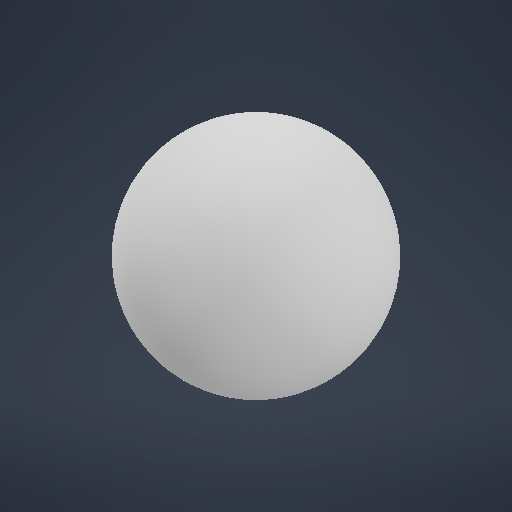
# Autodesk Inventor part: body
Saved by Autodesk Inventor 2026.1 (Build 301233000, 233)
## iProperties
Created: 2025-09-08
Part Number: body
Material: 일반
Document SubType Name: Modeling
Designer: ytw32
Density: 1 g/cm^3
Appearance: 기본값
Author: ytw32
Autodesk Inventor part; units mm, degrees
ref_plane "YZ Plane" through (0, 0, 0) normal (1, 0, 0) x (0, 1, 0)
ref_plane "XZ Plane" through (0, 0, 0) normal (0, 1, 0) x (-1, 0, 0)
ref_plane "XY Plane" through (0, 0, 0) normal (0, 0, 1) x (1, 0, 0)
sketch "스케치1" plane through (0, 0, 0) normal (0, 0, 1) x (1, 0, 0)
  arc A0 (0, 1500) -> (0, -1500) centre (0, 0) ccw
  line L0 (0, 1500) -> (0, -1500)
  dimension "d1" = 90
  constraints: 2 end point, 2 point on circle, 1 centre point, 1 coincident, 1 vertical
revolve "회전1" add sketch "스케치1" angle 360 about axis through (0, 1500, 0) along (0, -1, 0)
